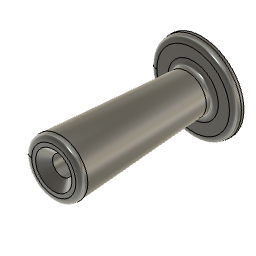
model (Autodesk Fusion 360 design; units mm, degrees)
Autodesk Fusion 360 part; units mm, degrees
sketch "Sketch1" plane through (0, 0, 0) normal (0, 1, 0) x (1, 0, 0)
  circle A0 centre (0, 0) radius 2.3
  circle A1 centre (0, 0) radius 4.35
  circle A2 centre (0, 0) radius 10
  dimension "d1" = 4.6
  dimension "d2" = 8.7
  dimension "d6" = 20
  constraint coincident A0.centre A1.centre
  constraint concentric A0 A2
  measures "d1" diameter of A0
  measures "d2" diameter of A1
  measures "d6" diameter of A2
extrude "Extrude1" add sketch "Sketch1" against normal blind 35 draft 3.8 contours A1
extrude "Extrude3" cut sketch "Sketch1" against normal up to surface (35 mm away) contours A0
chamfer "Chamfer1" distance 2 angle 45 1 edges at (-2.1444, -35, 0.8317)
extrude "Extrude2" add sketch "Sketch1" against normal blind 2 contours A2
fillet "Fillet1" chord length 2 tangency weight 2 3 edges at (-9.3233, -2, -3.6162) (-4.1795, -2, -1.6211) (-6.223, -35, 2.4137)
equation "d3 = -( 50 mm - 15 mm )"
